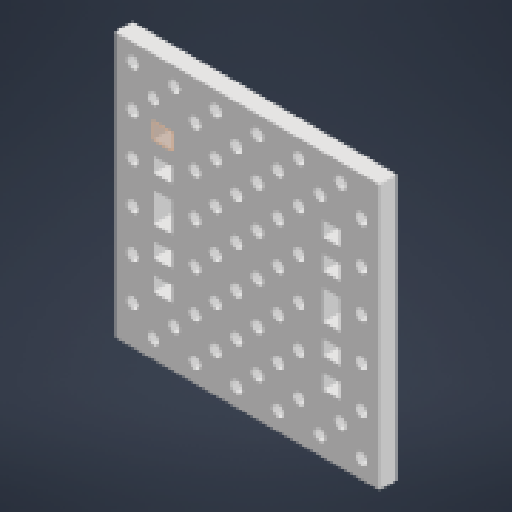
# Autodesk Inventor part: ScrewPlateLarge
Saved by Autodesk Inventor 2027 (Build 310192000, 192)
## iProperties
Created: 2026-04-15
Part Number: ScrewPlateLarge
Material: Generic
Document SubType Name: Modeling
Designer: Tueha
Density: 1 g/cm^3
Appearance: Default
Author: Tueha
Autodesk Inventor part; units mm, degrees
ref_plane "YZ Plane" through (0, 0, 0) normal (1, 0, 0) x (0, 1, 0)
ref_plane "XZ Plane" through (0, 0, 0) normal (0, 1, 0) x (-1, 0, 0)
ref_plane "XY Plane" through (0, 0, 0) normal (0, 0, 1) x (1, 0, 0)
ref_plane "Work Plane1" through (-28.4751, 43.9677, 58.8284) normal (0, 0, 1) x (1, 0, 0)
sketch "Sketch1" plane through (-28.4751, 43.9677, 58.8284) normal (0, 0, 1) x (1, 0, 0)
  line L0 (-16.2, 22.5) -> (73.8, 22.5)
  line L1 (73.8, 22.5) -> (73.8, -67.5)
  line L2 (73.8, -67.5) -> (-16.2, -67.5)
  line L3 (-16.2, -67.5) -> (-16.2, 22.5)
  line L4 (-3, -2.5) -> (3, -2.5) projected
  line L5 (3, -2.5) -> (3, 2.5) projected
  line L6 (3, 2.5) -> (-3, 2.5) projected
  line L7 (-3, 2.5) -> (-3, -2.5) projected
  line L8 (-3, -12.5) -> (3, -12.5) projected
  line L9 (3, -12.5) -> (3, -7.5) projected
  line L10 (3, -7.5) -> (-3, -7.5) projected
  line L11 (-3, -7.5) -> (-3, -12.5) projected
  line L12 (-3, -27.5) -> (3, -27.5) projected
  line L13 (3, -27.5) -> (3, -17.5) projected
  line L14 (3, -17.5) -> (-3, -17.5) projected
  line L15 (-3, -17.5) -> (-3, -27.5) projected
  line L16 (-3, -37.5) -> (3, -37.5) projected
  line L17 (3, -37.5) -> (3, -32.5) projected
  line L18 (3, -32.5) -> (-3, -32.5) projected
  line L19 (-3, -32.5) -> (-3, -37.5) projected
  line L20 (-3, -47.5) -> (3, -47.5) projected
  line L21 (3, -47.5) -> (3, -42.5) projected
  line L22 (3, -42.5) -> (-3, -42.5) projected
  line L23 (-3, -42.5) -> (-3, -47.5) projected
  line L24 (54.6, -47.5) -> (60.6, -47.5) projected
  line L25 (60.6, -47.5) -> (60.6, -42.5) projected
  line L26 (60.6, -42.5) -> (54.6, -42.5) projected
  line L27 (54.6, -42.5) -> (54.6, -47.5) projected
  line L28 (54.6, -32.5) -> (54.6, -37.5) projected
  line L29 (54.6, -37.5) -> (60.6, -37.5) projected
  line L30 (60.6, -37.5) -> (60.6, -32.5) projected
  line L31 (60.6, -32.5) -> (54.6, -32.5) projected
  line L32 (54.6, -32.5) -> (54.6, -37.5) projected
  line L33 (54.6, -27.5) -> (60.6, -27.5) projected
  line L34 (60.6, -27.5) -> (60.6, -17.5) projected
  line L35 (60.6, -17.5) -> (54.6, -17.5) projected
  line L36 (54.6, -17.5) -> (54.6, -27.5) projected
  line L37 (54.6, -12.5) -> (60.6, -12.5) projected
  line L38 (60.6, -12.5) -> (60.6, -7.5) projected
  line L39 (60.6, -7.5) -> (54.6, -7.5) projected
  line L40 (54.6, -7.5) -> (54.6, -12.5) projected
  line L41 (54.6, -2.5) -> (60.6, -2.5) projected
  line L42 (60.6, -2.5) -> (60.6, 2.5) projected
  line L43 (60.6, 2.5) -> (54.6, 2.5) projected
  line L44 (54.6, 2.5) -> (54.6, -2.5) projected
  point P0 (28.4751, -43.9677)
  point P1 (0, 2.5)
  point P2 (-3, 0)
  dimension "d0" = 90
  dimension "d1" = 90
  dimension "d2" = 20
  dimension "d3" = 13.2
  constraints: 8 end point, 2 midpoint, 2 parallel, 1 horizontal, 1 perpendicular
  measures "d0" distance of L1.end L2.end
  measures "d1" distance of L0.end L1.end
  measures "d2" distance from line of L0 point (0, 2.5)
  measures "d3" distance from line of L3 point (-3, 0)
extrude "Extrusion1" add sketch "Sketch1" against normal blind 6
sketch "Sketch2" plane through (-28.4751, 43.9677, 58.8284) normal (0, 0, 1) x (1, 0, 0)
  circle A0 centre (-10.2, 16.5) radius 2
  line L0 (73.8, 22.5) -> (-16.2, 22.5) projected
  line L1 (-16.2, 22.5) -> (-16.2, -67.5) projected
  line L2 (-16.2, 22.5) -> (73.8, -67.5)
  line L3 (73.8, 22.5) -> (-16.2, -67.5)
  circle A1 centre (-3.1289, 9.4289) radius 2
  circle A2 centre (3.9421, 2.3579) radius 2
  circle A3 centre (11.0132, -4.7132) radius 2
  circle A4 centre (18.0843, -11.7843) radius 2
  circle A5 centre (25.1553, -18.8553) radius 2
  circle A6 centre (32.2264, -25.9264) radius 2
  circle A7 centre (39.2975, -32.9975) radius 2
  circle A8 centre (46.3685, -40.0685) radius 2
  circle A9 centre (53.4396, -47.1396) radius 2
  circle A10 centre (60.5107, -54.2107) radius 2
  circle A11 centre (67.5817, -61.2817) radius 2
  circle A12 centre (-17.2711, 9.4289) radius 2
  circle A13 centre (-10.2, 2.3579) radius 2
  circle A14 centre (-3.1289, -4.7132) radius 2
  circle A15 centre (3.9421, -11.7843) radius 2
  circle A16 centre (11.0132, -18.8553) radius 2
  circle A17 centre (18.0843, -25.9264) radius 2
  circle A18 centre (25.1553, -32.9975) radius 2
  circle A19 centre (32.2264, -40.0685) radius 2
  circle A20 centre (39.2975, -47.1396) radius 2
  circle A21 centre (46.3685, -54.2107) radius 2
  circle A22 centre (53.4396, -61.2817) radius 2
  circle A23 centre (60.5107, -68.3528) radius 2
  circle A24 centre (-3.1289, 23.5711) radius 2
  circle A25 centre (3.9421, 16.5) radius 2
  circle A26 centre (11.0132, 9.4289) radius 2
  circle A27 centre (18.0843, 2.3579) radius 2
  circle A28 centre (25.1553, -4.7132) radius 2
  circle A29 centre (32.2264, -11.7843) radius 2
  circle A30 centre (39.2975, -18.8553) radius 2
  circle A31 centre (46.3685, -25.9264) radius 2
  circle A32 centre (53.4396, -32.9975) radius 2
  circle A33 centre (60.5107, -40.0685) radius 2
  circle A34 centre (67.5817, -47.1396) radius 2
  circle A35 centre (74.6528, -54.2107) radius 2
  circle A36 centre (-24.3421, 2.3579) radius 2
  circle A37 centre (-17.2711, -4.7132) radius 2
  circle A38 centre (-10.2, -11.7843) radius 2
  circle A39 centre (-3.1289, -18.8553) radius 2
  circle A40 centre (3.9421, -25.9264) radius 2
  circle A41 centre (11.0132, -32.9975) radius 2
  circle A42 centre (18.0843, -40.0685) radius 2
  circle A43 centre (25.1553, -47.1396) radius 2
  circle A44 centre (32.2264, -54.2107) radius 2
  circle A45 centre (39.2975, -61.2817) radius 2
  circle A46 centre (46.3685, -68.3528) radius 2
  circle A47 centre (53.4396, -75.4239) radius 2
  circle A48 centre (3.9421, 30.6421) radius 2
  circle A49 centre (11.0132, 23.5711) radius 2
  circle A50 centre (18.0843, 16.5) radius 2
  circle A51 centre (25.1553, 9.4289) radius 2
  circle A52 centre (32.2264, 2.3579) radius 2
  circle A53 centre (39.2975, -4.7132) radius 2
  circle A54 centre (46.3685, -11.7843) radius 2
  circle A55 centre (53.4396, -18.8553) radius 2
  circle A56 centre (60.5107, -25.9264) radius 2
  circle A57 centre (67.5817, -32.9975) radius 2
  circle A58 centre (74.6528, -40.0685) radius 2
  circle A59 centre (81.7239, -47.1396) radius 2
  circle A60 centre (-31.4132, -4.7132) radius 2
  circle A61 centre (-24.3421, -11.7843) radius 2
  circle A62 centre (-17.2711, -18.8553) radius 2
  circle A63 centre (-10.2, -25.9264) radius 2
  circle A64 centre (-3.1289, -32.9975) radius 2
  circle A65 centre (3.9421, -40.0685) radius 2
  circle A66 centre (11.0132, -47.1396) radius 2
  circle A67 centre (18.0843, -54.2107) radius 2
  circle A68 centre (25.1553, -61.2817) radius 2
  circle A69 centre (32.2264, -68.3528) radius 2
  circle A70 centre (39.2975, -75.4239) radius 2
  circle A71 centre (46.3685, -82.4949) radius 2
  circle A72 centre (11.0132, 37.7132) radius 2
  circle A73 centre (18.0843, 30.6421) radius 2
  circle A74 centre (25.1553, 23.5711) radius 2
  circle A75 centre (32.2264, 16.5) radius 2
  circle A76 centre (39.2975, 9.4289) radius 2
  circle A77 centre (46.3685, 2.3579) radius 2
  circle A78 centre (53.4396, -4.7132) radius 2
  circle A79 centre (60.5107, -11.7843) radius 2
  circle A80 centre (67.5817, -18.8553) radius 2
  circle A81 centre (74.6528, -25.9264) radius 2
  circle A82 centre (81.7239, -32.9975) radius 2
  circle A83 centre (88.7949, -40.0685) radius 2
  circle A84 centre (-38.4843, -11.7843) radius 2
  circle A85 centre (-31.4132, -18.8553) radius 2
  circle A86 centre (-24.3421, -25.9264) radius 2
  circle A87 centre (-17.2711, -32.9975) radius 2
  circle A88 centre (-10.2, -40.0685) radius 2
  circle A89 centre (-3.1289, -47.1396) radius 2
  circle A90 centre (3.9421, -54.2107) radius 2
  circle A91 centre (11.0132, -61.2817) radius 2
  circle A92 centre (18.0843, -68.3528) radius 2
  circle A93 centre (25.1553, -75.4239) radius 2
  circle A94 centre (32.2264, -82.4949) radius 2
  circle A95 centre (39.2975, -89.566) radius 2
  circle A96 centre (18.0843, 44.7843) radius 2
  circle A97 centre (25.1553, 37.7132) radius 2
  circle A98 centre (32.2264, 30.6421) radius 2
  circle A99 centre (39.2975, 23.5711) radius 2
  circle A100 centre (46.3685, 16.5) radius 2
  circle A101 centre (53.4396, 9.4289) radius 2
  circle A102 centre (60.5107, 2.3579) radius 2
  circle A103 centre (67.5817, -4.7132) radius 2
  circle A104 centre (74.6528, -11.7843) radius 2
  circle A105 centre (81.7239, -18.8553) radius 2
  circle A106 centre (88.7949, -25.9264) radius 2
  circle A107 centre (95.866, -32.9975) radius 2
  circle A108 centre (-45.5553, -18.8553) radius 2
  circle A109 centre (-38.4843, -25.9264) radius 2
  circle A110 centre (-31.4132, -32.9975) radius 2
  circle A111 centre (-24.3421, -40.0685) radius 2
  circle A112 centre (-17.2711, -47.1396) radius 2
  circle A113 centre (-10.2, -54.2107) radius 2
  circle A114 centre (-3.1289, -61.2817) radius 2
  circle A115 centre (3.9421, -68.3528) radius 2
  circle A116 centre (11.0132, -75.4239) radius 2
  circle A117 centre (18.0843, -82.4949) radius 2
  circle A118 centre (25.1553, -89.566) radius 2
  circle A119 centre (32.2264, -96.6371) radius 2
  circle A120 centre (25.1553, 51.8553) radius 2
  circle A121 centre (32.2264, 44.7843) radius 2
  circle A122 centre (39.2975, 37.7132) radius 2
  circle A123 centre (46.3685, 30.6421) radius 2
  circle A124 centre (53.4396, 23.5711) radius 2
  circle A125 centre (60.5107, 16.5) radius 2
  circle A126 centre (67.5817, 9.4289) radius 2
  circle A127 centre (74.6528, 2.3579) radius 2
  circle A128 centre (81.7239, -4.7132) radius 2
  circle A129 centre (88.7949, -11.7843) radius 2
  circle A130 centre (95.866, -18.8553) radius 2
  circle A131 centre (102.9371, -25.9264) radius 2
  circle A132 centre (-52.6264, -25.9264) radius 2
  circle A133 centre (-45.5553, -32.9975) radius 2
  circle A134 centre (-38.4843, -40.0685) radius 2
  circle A135 centre (-31.4132, -47.1396) radius 2
  circle A136 centre (-24.3421, -54.2107) radius 2
  circle A137 centre (-17.2711, -61.2817) radius 2
  circle A138 centre (-10.2, -68.3528) radius 2
  circle A139 centre (-3.1289, -75.4239) radius 2
  circle A140 centre (3.9421, -82.4949) radius 2
  circle A141 centre (11.0132, -89.566) radius 2
  circle A142 centre (18.0843, -96.6371) radius 2
  circle A143 centre (25.1553, -103.7082) radius 2
  point P0 (28.4751, -43.9677)
  dimension "d6" = 4
  dimension "d7" = 6
  dimension "d8" = 6
  dimension "d11" = 10
  dimension "d14" = 10
  constraints: 144 centre point, 4 end point, 288 other
  measures "d6" diameter of A0
  measures "d7" distance from line of L0 A0.centre
  measures "d8" distance from line of L1 A0.centre
  measures "d11" distance of A0.centre A1.centre
  measures "d14" distance of A0.centre A12.centre
extrude "Extrusion2" cut sketch "Sketch2" against normal blind 6 contours A0 L2 | L2 A0 | A11 L2 | L2 A11 | A10 L2 | L2 A10 | A8 L2 | L2 A8 | A7 L2 | L2 A7 | A6 L2 | L2 A6 | A1 L2 | L2 A1 | A3 L2 | L2 A3 | A4 L2 | L2 A4 | A5 L2 | L2 A5 | A13 | A16 | A17 | A18 | A19 | A20 | A21 | A22 | A25 | A26 | A27 | A28 | A29 | A30 | A31 | A34 | A38 | A41 | A42 | A43 | A44 | A45 | A50 | A51 | A52 | A53 | A54 | A57 | A63 | A66 | A67 | A68 | A75 | A76 | A77 | A80 | A88 | A90 | A91 | A100 | A101 | A103 | A113 | A114 | A125 | A126
body "Solid1"
